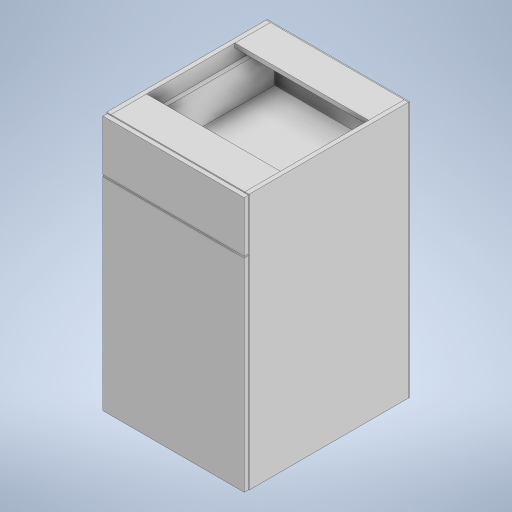
# Autodesk Inventor part: Base Cabinet 2
Saved by Autodesk Inventor 2024 (Build 280153000, 153)
## iProperties
Created: 2023-06-24
Part Number: Base Cabinet 2
Material: Generic
Document SubType Name: Modeling
Designer: 69
Density: 1 g/cm^3
Appearance: Default
Author: 69
Autodesk Inventor part; units mm, degrees
sketch "Sketch1" plane through (0, 0, 0) normal (0, 0, 1) x (1, 0, 0)
  line L0 (-1498, 0) -> (1498, 0) construction
  line L1 (-1498, 0) -> (-898, 0)
  line L2 (-898, 0) -> (-898, 2068)
  line L3 (-898, 2068) -> (-1498, 2068)
  line L4 (-1498, 2068) -> (-1498, 0)
  line L5 (-898, 0) -> (-498, 0)
  line L6 (-498, 0) -> (-498, 816)
  line L7 (-498, 816) -> (-898, 816)
  line L8 (-898, 816) -> (-898, 0)
  line L9 (-498, 0) -> (102, 0)
  line L10 (102, 0) -> (102, 816)
  line L11 (102, 816) -> (-498, 816)
  line L12 (-498, 816) -> (-498, 0)
  line L13 (102, 0) -> (698, 0)
  line L14 (698, 0) -> (698, 668)
  line L15 (698, 668) -> (102, 668)
  line L16 (102, 668) -> (102, 0)
  line L17 (698, 0) -> (1498, 0)
  line L18 (1498, 0) -> (1498, 816)
  line L19 (1498, 816) -> (698, 816)
  line L20 (698, 816) -> (698, 0)
  line L21 (-1498, 0) -> (1498, 0)
  line L22 (1498, 0) -> (1498, 96)
  line L23 (1498, 96) -> (-1498, 96)
  line L24 (-1498, 96) -> (-1498, 0)
  line L25 (-898, 816) -> (1498, 816)
  line L26 (1498, 816) -> (1498, 832)
  line L27 (1498, 832) -> (-898, 832)
  line L28 (-898, 832) -> (-898, 816)
  line L29 (-898, 1972) -> (-498, 1972)
  line L30 (-498, 1972) -> (-498, 1372)
  line L31 (-498, 1372) -> (-898, 1372)
  line L32 (-898, 1372) -> (-898, 1972)
  line L33 (698, 1972) -> (1498, 1972)
  line L34 (1498, 1972) -> (1498, 1372)
  line L35 (1498, 1372) -> (698, 1372)
  line L36 (698, 1372) -> (698, 1972)
  line L37 (698, 1372) -> (98, 1372)
  line L38 (98, 1372) -> (98, 1972)
  line L39 (98, 1972) -> (698, 1972)
  line L40 (698, 1972) -> (698, 1372)
  line L41 (-498, 1372) -> (98, 1372)
  line L42 (-498, 1372) -> (-275, 1637.7611)
  line L43 (98, 1372) -> (-125, 1637.7611)
  line L44 (-275, 1637.7611) -> (-125, 1637.7611)
  line L45 (-125, 1637.7611) -> (-125, 2068)
  line L46 (-125, 2068) -> (-275, 2068)
  line L47 (-275, 2068) -> (-275, 1637.7611)
  line L48 (1098, 816) -> (1098, 96)
  line L49 (-198, 816) -> (-198, 96)
  line L50 (-898, 668) -> (-498, 668)
  line L51 (-1498, 520) -> (-898, 520)
  line L52 (-1498, 1579) -> (-898, 1579)
  line L53 (398, 1972) -> (398, 1372)
  line L54 (1098, 1972) -> (1098, 1372)
  line L55 (698, 1876) -> (1498, 1876)
  line L56 (698, 1468) -> (1498, 1468)
  line L57 (-1498, 1049.5) -> (-898, 1049.5)
  point P0 (0, 0)
  point P1 (0, 0)
  point P2 (0, 0)
  point P3 (-198, 816)
  point P4 (0, 0)
  dimension "d0" = 2996
  dimension "d1" = 600
  dimension "d2" = 2068
  dimension "d3" = 400
  dimension "d4" = 816
  dimension "d5" = 600
  dimension "d6" = 816
  dimension "d7" = 596
  dimension "d8" = 668
  dimension "d9" = 800
  dimension "d10" = 816
  dimension "d11" = 96
  dimension "d12" = 16
  dimension "d13" = 400
  dimension "d14" = 600
  dimension "d15" = 96
  dimension "d16" = 800
  dimension "d17" = 600
  dimension "d18" = 600
  dimension "d19" = 600
  dimension "d20" = 50
  dimension "d21" = 150
  dimension "d22" = 148
  dimension "d23" = 1059
  dimension "d24" = 96
  dimension "d25" = 96
  dimension "d26" = 529.5
  constraints: 116 end point, 22 parallel, 18 point on line, 17 perpendicular, 14 horizontal, 8 midpoint, 4 coincident, 4 horizontal alignment, 2 vertical alignment, 1 equal length
  measures "d0" distance of L0.start L0.end
  measures "d1" distance of L3.end L2.end
  measures "d2" distance of L2.end L1.end
  measures "d3" distance of L7.end L6.end
  measures "d4" distance of L6.end L5.end
  measures "d5" distance of L11.end L10.end
  measures "d6" distance of L9.end L10.end
  measures "d7" distance of L15.end L14.end
  measures "d8" distance of L14.end L13.end
  measures "d9" distance of L19.end L18.end
  measures "d10" distance of L18.end L17.end
  measures "d11" distance of L22.end L21.end
  measures "d12" distance of L26.end L25.end
  measures "d13" distance of L30.end L31.end
  measures "d14" distance of L29.end L30.end
  measures "d15" distance between parallel lines of L3 L29
  measures "d16" distance of L34.end L35.end
  measures "d17" distance of L33.end L34.end
  measures "d18" distance of L38.end L39.end
  measures "d19" distance of L37.end L38.end
  measures "d20" angle of L41 L42
  measures "d21" distance of L43.end L42.end
  measures "d22" distance of L50.start L51.end
  measures "d23" distance between parallel lines of L51 L52
  measures "d24" distance of L33.start L55.start
  measures "d25" distance of L56.start L35.end
  measures "d26" distance between parallel lines of L51 L57
ref_plane "Work Plane1" through (1498, 96, 0) normal (0, 1, 0) x (-1, 0, 0)
sketch "Sketch2" plane through (1498, 96, 0) normal (0, 1, 0) x (-1, 0, 0)
  line L0 (2396, 0) -> (1996, 0)
  line L1 (1996, 0) -> (1996, 460)
  line L2 (1996, 460) -> (2396, 460)
  line L3 (2396, 460) -> (2396, 0)
  line L4 (2384, 12) -> (2008, 12)
  line L5 (2008, 12) -> (2008, 448)
  line L6 (2008, 448) -> (2384, 448)
  line L7 (2384, 448) -> (2384, 12)
  line L8 (2384, 12) -> (2384, 0)
  line L9 (2008, 12) -> (2008, 0)
  line L10 (2384, 448) -> (2396, 448)
  line L11 (2008, 448) -> (1996, 448)
  point P0 (1498, 0)
  point P1 (1996, 0)
  point P2 (2396, 0)
  dimension "d28" = 460
  dimension "d29" = 12
  constraints: 24 end point, 6 perpendicular, 4 parallel, 4 point on line, 1 coincident, 1 horizontal, 3 other
  measures "d28" distance of L0.end L1.end
  measures "d29" distance between parallel lines of L3 L7
extrude "Extrusion1" add sketch "Sketch2" along normal up to surface (720 mm away) contours L0 L8 L7 L10 L3 | L0 L1 L11 L5 L9
extrude "Extrusion2" add sketch "Sketch2" along normal up to surface (720 mm away) separate body contours L10 L6 L11 L1 L2 L3
split body "Split1" sketch "Sketch1" result two bodies bodies 2 curves L50 first body at (-764.6667, 717.3333, 459.5)
sketch "Sketch3" plane through (1498, 96, 0) normal (0, 1, 0) x (-1, 0, 0)
  line L0 (2396, 0) -> (1996, 0)
  line L1 (1996, 0) -> (1996, -3)
  line L2 (1996, -3) -> (2396, -3)
  line L3 (2396, -3) -> (2396, 0)
  point P0 (1498, 0)
  dimension "d34" = 3
  constraints: 8 end point, 2 parallel, 1 coincident, 1 horizontal, 1 perpendicular
  measures "d34" distance of L2.end L0.start
extrude "Extrusion3" add sketch "Sketch3" along normal up to surface (720 mm away) separate body
sketch "Sketch4" plane through (1498, 96, 0) normal (0, 1, 0) x (-1, 0, 0)
  line L0 (1996, 0) -> (2396, 0) projected
  line L1 (2384, 0) -> (2384, 448) projected
  line L2 (2008, 448) -> (2008, 0) projected
  line L3 (2396, 448) -> (1996, 448) projected
  point P0 (1498, 0)
extrude "Extrusion4" add sketch "Sketch4" along normal blind 12 separate body
ref_plane "Work Plane2" through (-898, 816, 112) normal (0, -1, 0) x (0, 0, -1)
sketch "Sketch5" plane through (-898, 816, 112) normal (0, -1, 0) x (0, 0, -1)
  line L0 (-336, 0) -> (-336, 400) projected
  line L1 (112, 12) -> (-336, 12) projected
  line L2 (-336, 388) -> (112, 388) projected
  line L3 (-236, 12) -> (-236, 388)
  line L4 (12, 12) -> (12, 388)
  line L5 (112, 400) -> (112, 0) projected
  point P0 (112, 898)
  dimension "d39" = 100
  dimension "d40" = 100
  constraints: 4 end point, 4 point on line, 2 perpendicular
  measures "d39" distance between parallel lines of L0 L3
  measures "d40" distance between parallel lines of L5 L4
extrude "Extrusion5" add sketch "Sketch5" along normal blind 12 separate body contours L0 L2 L3 L1 | L4 L2 L5 L1
sketch "Sketch6" plane through (-898, 96, 460) normal (0, 0, 1) x (1, 0, 0)
  line L0 (0, 0) -> (0, 720) projected
  line L1 (400, 0) -> (400, 720) projected
  line L2 (0, 573.5) -> (400, 573.5)
  line L3 (400, 573.5) -> (400, 570.5)
  line L4 (400, 570.5) -> (0, 570.5)
  line L5 (0, 570.5) -> (0, 573.5)
  line L6 (400, 572) -> (0, 572) projected
  point P0 (898, -96)
  point P1 (0, 570.5)
  dimension "d43" = 1.5
  dimension "d44" = 1.5
  constraints: 8 end point, 2 parallel, 2 point on line, 1 horizontal, 1 perpendicular
  measures "d43" distance between parallel lines of L6 L2
  measures "d44" distance between parallel lines of L6 L4
extrude "Extrusion6" cut sketch "Sketch6" against normal blind 12 bodies 3 4
ref_plane "Work Plane4" through (-498, 681.5, 460) normal (0, 1, 0) x (0, 0, -1)
ref_plane "Work Plane3" through (-498, 669.5, 460) normal (0, 1, 0) x (0, 0, -1)
sketch "Sketch7" plane through (-498, 681.5, 460) normal (0, 1, 0) x (0, 0, -1)
  line L0 (460, 0) -> (460, 400) projected
  line L1 (460, 388) -> (12, 388) projected
  line L2 (12, 12) -> (460, 12) projected
  line L3 (12, 400) -> (12, 0) projected
  line L4 (460, 388) -> (12, 12) construction
  line L5 (448, 376) -> (24, 376)
  line L6 (24, 376) -> (24, 24)
  line L7 (24, 24) -> (448, 24)
  line L8 (448, 24) -> (448, 376)
  line L9 (448, 376) -> (24, 24) construction
  line L10 (24, 376) -> (448, 24) construction
  line L11 (24, 376) -> (12, 376)
  line L12 (24, 24) -> (12, 24)
  line L13 (24, 364) -> (436, 364)
  line L14 (436, 364) -> (436, 36)
  line L15 (436, 36) -> (24, 36)
  line L16 (24, 364) -> (12, 364)
  line L17 (24, 36) -> (12, 36)
  line L18 (436, 364) -> (448, 364)
  line L19 (436, 36) -> (448, 36)
  point P0 (460, -498)
  point P1 (236, 200)
  dimension "d48" = 12
  dimension "d49" = 12
  dimension "d50" = 12
  constraints: 32 end point, 8 point on line, 4 perpendicular, 3 midpoint, 3 parallel, 2 horizontal, 2 other
  measures "d48" distance between parallel lines of L0 L8
  measures "d49" distance between parallel lines of L2 L7
  measures "d50" distance between parallel lines of L8 L14
extrude "Extrusion7" add sketch "Sketch7" along normal blind 100 separate body contours L3 L17 L6 L12 | L11 L6 L16 L3 | L6 L15 L19 L8 L7 | L5 L8 L18 L13 L6
sketch "Sketch8" plane through (-498, 681.5, 460) normal (0, 1, 0) x (0, 0, -1)
  line L0 (448, 376) -> (451, 376)
  line L1 (451, 376) -> (451, 24)
  line L2 (451, 24) -> (448, 24)
  line L3 (448, 24) -> (448, 376)
  point P0 (460, -498)
  dimension "d53" = 3
  constraints: 8 end point, 2 parallel, 1 coincident, 1 horizontal, 1 perpendicular
  measures "d53" distance of L1.end L2.end
extrude "Extrusion8" add sketch "Sketch8" along normal up to surface (100 mm away) separate body
sketch "Sketch9" plane through (-498, 681.5, 460) normal (0, 1, 0) x (0, 0, -1)
  line L0 (451, 24) -> (451, 376) projected
  line L1 (12, 0) -> (12, 400) projected
  line L2 (451, 24) -> (12, 24)
  line L3 (12, 24) -> (12, 376)
  line L4 (12, 376) -> (451, 376)
  line L5 (451, 376) -> (451, 24)
  point P0 (460, -498)
  constraints: 8 end point, 2 parallel, 1 horizontal, 1 perpendicular, 1 point on line
extrude "Extrusion9" add sketch "Sketch9" against normal blind 3 separate body
sketch "Sketch10" plane through (-898, 96, 0) normal (0, 0, 1) x (1, 0, 0)
  line L0 (12, 0) -> (12, 720) projected
  line L1 (388, 0) -> (388, 720) projected
  line L2 (12, 302) -> (388, 302)
  line L3 (388, 302) -> (388, 290)
  line L4 (388, 290) -> (12, 290)
  line L5 (12, 290) -> (12, 302)
  line L6 (12, 0) -> (388, 0) projected
  point P0 (898, -96)
  point P1 (12, 290)
  dimension "d58" = 290
  dimension "d59" = 12
  constraints: 8 end point, 2 parallel, 2 point on line, 1 horizontal, 1 perpendicular
  measures "d58" distance between parallel lines of L6 L4
  measures "d59" distance between parallel lines of L4 L2
extrude "Extrusion10" add sketch "Sketch10" along normal up to surface (448 mm away) separate body contours L0 L2 L1 L4
sketch "Sketch12" plane through (-898, 816, 460) normal (0, 0, 1) x (1, 0, 0)
  line L0 (0, -720) -> (0, 0) projected
  line L1 (400, -720) -> (400, 0) projected
  line L2 (0, 0) -> (400, 0)
  line L3 (400, 0) -> (400, -3)
  line L4 (400, -3) -> (0, -3)
  line L5 (0, -3) -> (0, 0)
  line L6 (0, -720) -> (400, -720) projected
  line L7 (0, -3) -> (1.5, -3)
  line L8 (1.5, -3) -> (1.5, -720)
  line L9 (1.5, -720) -> (0, -720)
  line L10 (0, -720) -> (0, -3)
  line L11 (400, -3) -> (398.5, -3)
  line L12 (398.5, -3) -> (398.5, -720)
  line L13 (398.5, -720) -> (400, -720)
  line L14 (400, -720) -> (400, -3)
  point P0 (898, -816)
  point P1 (1.5, -3)
  dimension "d66" = 3
  dimension "d67" = 1.5
  dimension "d68" = 1.5
  constraints: 24 end point, 6 parallel, 3 horizontal, 3 perpendicular, 3 point on line
  measures "d66" distance of L1.end L3.end
  measures "d67" distance of L1.start L12.end
  measures "d68" distance of L8.end L0.start
extrude "Extrusion12" cut sketch "Sketch12" against normal blind 12 contours L0 L4 L8 L6 | L0 L2 L1 L4 | L12 L4 L1 L6 bodies 3 4
